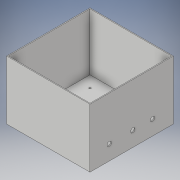
# Autodesk Inventor part: 546-1550Z137-Combiner
Saved by Autodesk Inventor 2018 (Build 220112000, 112)
## iProperties
Created: 2018-04-30
Part Number: 546-1550Z137-Combiner
Material: Generic
Document SubType Name: Modeling
Designer: bbramman
Density: 1 g/cm^3
Appearance: Default
Author: bbramman
Autodesk Inventor part; units mm, degrees
ref_plane "YZ Plane" through (0, 0, 0) normal (1, 0, 0) x (0, 1, 0)
ref_plane "XZ Plane" through (0, 0, 0) normal (0, 1, 0) x (-1, 0, 0)
ref_plane "XY Plane" through (0, 0, 0) normal (0, 0, 1) x (1, 0, 0)
sketch "Sketch1" plane through (0, 0, 0) normal (0, 1, 0) x (-1, 0, 0)
  line L0 (-60.452, -60.452) -> (60.452, -60.452)
  line L1 (60.452, -60.452) -> (60.452, 60.452)
  line L2 (60.452, 60.452) -> (-60.452, 60.452)
  line L3 (-60.452, 60.452) -> (-60.452, -60.452)
  line L4 (-60.452, -60.452) -> (60.452, 60.452) construction
  line L5 (60.452, -60.452) -> (-60.452, 60.452) construction
  point P0 (0, 0)
  dimension "d0" = 120.904
  dimension "d1" = 120.904
  constraints: 12 end point, 2 midpoint, 2 parallel, 1 horizontal, 1 perpendicular
  measures "d0" distance of L2.end L1.end
  measures "d1" distance of L1.end L0.end
extrude "Extrusion1" add sketch "Sketch1" along normal blind 2.54
sketch "Sketch2" plane through (0, 2.54, 0) normal (0, 1, 0) x (1, 0, 0)
  line L0 (60.452, 60.452) -> (-60.452, 60.452) projected
  line L1 (60.452, -60.452) -> (-60.452, -60.452)
  line L2 (-60.452, -60.452) -> (-60.452, 60.452)
  line L3 (-60.452, 60.452) -> (60.452, 60.452)
  line L4 (60.452, 60.452) -> (60.452, -60.452)
  line L5 (60.452, -60.452) -> (-60.452, 60.452) construction
  line L6 (-60.452, -60.452) -> (60.452, 60.452) construction
  line L7 (59.182, -59.182) -> (-59.182, -59.182)
  line L8 (-59.182, -59.182) -> (-59.182, 59.182)
  line L9 (-59.182, 59.182) -> (59.182, 59.182)
  line L10 (59.182, 59.182) -> (59.182, -59.182)
  line L11 (59.182, -59.182) -> (-59.182, 59.182) construction
  line L12 (-59.182, -59.182) -> (59.182, 59.182) construction
  point P0 (0, 0)
  dimension "d4" = 118.364
  dimension "d5" = 118.364
  constraints: 24 end point, 4 midpoint, 4 parallel, 2 horizontal, 2 perpendicular
  measures "d4" distance of L8.end L9.end
  measures "d5" distance of L7.end L8.end
extrude "Extrusion2" add sketch "Sketch2" along normal blind 82.804
sketch "Sketch3" plane through (0, 2.54, 0) normal (0, 1, 0) x (1, 0, 0)
  circle A0 centre (0, -25.4) radius 2.0828
  circle A1 centre (0, 25.4) radius 2.0828
  point P0 (0, 0)
  dimension "d10" = 4.1656
  dimension "d11" = 4.1656
  constraints: 2 centre point
  measures "d10" diameter of A0
  measures "d11" diameter of A1
extrude "Extrusion3" cut sketch "Sketch3" against normal through all
sketch "Sketch4" plane through (0, 2.54, 0) normal (0, 1, 0) x (1, 0, 0)
  line L0 (32.9946, -9.9949) -> (-32.9946, 9.9949) construction
  line L1 (-32.9946, -9.9949) -> (32.9946, 9.9949) construction
  circle A0 centre (-32.9946, -9.9949) radius 1.4986
  circle A1 centre (-32.9946, 9.9949) radius 1.4986
  circle A2 centre (32.9946, -9.9949) radius 1.4986
  circle A3 centre (32.9946, 9.9949) radius 1.4986
  line L2 (50, -50) -> (-50, 50) construction
  line L3 (-50, -50) -> (50, 50) construction
  circle A4 centre (43.65, -42.38) radius 1.4224
  circle A5 centre (43.65, 42.38) radius 1.4224
  circle A6 centre (-42.38, 42.38) radius 1.4224
  circle A7 centre (-42.38, -42.38) radius 1.4224
  point P0 (0, 0)
  dimension "d14" = 65.9892
  dimension "d15" = 19.9898
  dimension "d16" = 2.9972
  dimension "d17" = 2.9972
  dimension "d18" = 2.9972
  dimension "d19" = 2.9972
  dimension "d20" = 100
  dimension "d21" = 100
  dimension "d28" = 2.8448
  dimension "d29" = 2.8448
  dimension "d30" = 2.8448
  dimension "d31" = 2.8448
  constraints: 8 centre point, 8 end point, 4 coincident, 4 midpoint
  measures "d14" distance of L0.end L1.end
  measures "d15" distance of L1.start L0.end
  measures "d16" diameter of A0
  measures "d17" diameter of A1
  measures "d18" diameter of A2
  measures "d19" diameter of A3
  measures "d20" distance of L2.end L3.end
  measures "d21" distance of L3.start L2.end
  measures "d28" diameter of A4
  measures "d29" diameter of A5
  measures "d30" diameter of A6
  measures "d31" diameter of A7
extrude "Extrusion4" cut sketch "Sketch4" against normal through all
sketch "Sketch5" plane through (-59.182, 2.54, 59.182) normal (1, 0, 0) x (0, 0, -1)
  line L0 (0, 0) -> (0, 82.804) projected
  circle A0 centre (59.182, 19.05) radius 3.175
  point P0 (59.182, -2.54)
  dimension "d34" = 6.35
  constraints: 1 centre point
  measures "d34" diameter of A0
extrude "Extrusion5" cut sketch "Sketch5" against normal through all
sketch "Sketch6" plane through (59.182, 2.54, -59.182) normal (-1, 0, 0) x (0, 0, 1)
  point P0 (59.182, -2.54)
sketch "Sketch7" plane through (59.182, 2.54, -59.182) normal (-1, 0, 0) x (0, 0, 1)
  circle A0 centre (29.0271, 19.05) radius 3.175
  circle A1 centre (57.6021, 19.05) radius 3.175
  circle A2 centre (91.7334, 19.05) radius 3.175
  point P0 (59.182, -2.54)
  dimension "d40" = 6.35
  dimension "d41" = 6.35
  dimension "d42" = 6.35
  constraints: 3 centre point
  measures "d40" diameter of A0
  measures "d41" diameter of A1
  measures "d42" diameter of A2
extrude "Extrusion6" cut sketch "Sketch7" against normal through all
body "Solid1"
